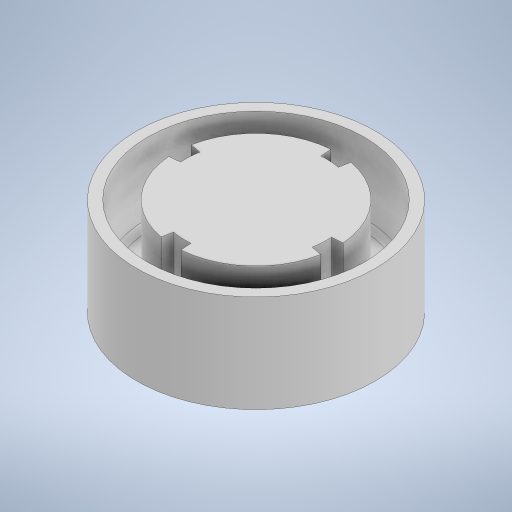
# Autodesk Inventor part: forma
Saved by Autodesk Inventor 2023.5 (Build 275446000, 446)
## iProperties
Created: 2025-03-27
Part Number: forma
Material: Ogólny
Document SubType Name: Modeling
Designer: kamil
Density: 1 g/cm^3
Appearance: Domyślna
Author: kamil
Autodesk Inventor part; units mm, degrees
ref_plane "YZ Plane" through (0, 0, 0) normal (1, 0, 0) x (0, 1, 0)
ref_plane "XZ Plane" through (0, 0, 0) normal (0, 1, 0) x (-1, 0, 0)
ref_plane "XY Plane" through (0, 0, 0) normal (0, 0, 1) x (1, 0, 0)
sketch "Szkic1" plane through (0, 0, 0) normal (0, 1, 0) x (-1, 0, 0)
  circle A0 centre (0, 0) radius 10
  circle A1 centre (0, 0) radius 11
  dimension "d0" = 20
  dimension "d1" = 1
  constraints: 2 centre point, 1 coincident
  measures "d0" diameter of A0
  measures "d1" radial gap between concentric circles of A0 A1
extrude "Wyciągnięcie proste1" add sketch "Szkic1" along normal blind 7
extrude "Wyciągnięcie proste2" add sketch "Szkic1" against normal blind 2 contours A0 | A1
sketch "Szkic2" plane through (0, 0, 0) normal (0, 1, 0) x (1, 0, 0)
  circle A0 centre (0, 0) radius 10 projected
  circle A1 centre (0, 0) radius 1.5
  line L0 (-1.3953, -7.3691) -> (-1.2093, -6.3865)
  arc A2 (-1.2093, -6.3865) -> (0.4849, -6.4819) centre (0, 0) ccw
  line L1 (0.4849, -6.4819) -> (0.5595, -7.4791)
  arc A3 (0.5595, -7.4791) -> (7.3691, -1.3953) centre (0, 0) ccw
  line L2 (7.3691, -1.3953) -> (6.3865, -1.2093)
  arc A4 (6.3865, -1.2093) -> (6.4819, 0.4849) centre (0, 0) ccw
  line L3 (6.4819, 0.4849) -> (7.4791, 0.5595)
  arc A5 (7.4791, 0.5595) -> (1.3953, 7.3691) centre (0, 0) ccw
  line L4 (1.3953, 7.3691) -> (1.2093, 6.3865)
  arc A6 (1.2093, 6.3865) -> (-0.4849, 6.4819) centre (0, 0) ccw
  line L5 (-0.4849, 6.4819) -> (-0.5595, 7.4791)
  arc A7 (-0.5595, 7.4791) -> (-7.3691, 1.3953) centre (0, 0) ccw
  line L6 (-7.3691, 1.3953) -> (-6.3865, 1.2093)
  arc A8 (-6.3865, 1.2093) -> (-6.4819, -0.4849) centre (0, 0) ccw
  line L7 (-6.4819, -0.4849) -> (-7.4791, -0.5595)
  arc A9 (-7.4791, -0.5595) -> (-1.3953, -7.3691) centre (0, 0) ccw
  point P0 (10.4507, -2.3919)
  constraints: 16 end point, 16 point on circle, 9 centre point
extrude "Wyciągnięcie proste3" add sketch "Szkic2" along normal blind 7 contours A1 | A9 L7 A8 L6 A7 L5 A6 L4 A5 L3 A4 L2 A3 L1 A2 L0
fillet "Zaokrąglenie1" radius 0.5 1 edges at (10, 0, 0)
